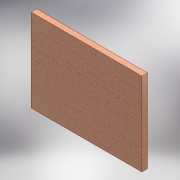
# Autodesk Inventor part: WoodBase
Saved by Autodesk Inventor 2018.2 (Build 222227000, 227)
## iProperties
Created: 2018-03-28
Part Number: WoodBase
Material: Wood (Oak)
Document SubType Name: Modeling
Designer: Muchen He
Density: 0.76 g/cm^3
Appearance: White Oak - Natural Medium Gloss
Author: Muchen He
Autodesk Inventor part; units mm, degrees
ref_plane "YZ Plane" through (0, 0, 0) normal (1, 0, 0) x (0, 1, 0)
ref_plane "XZ Plane" through (0, 0, 0) normal (0, 1, 0) x (-1, 0, 0)
ref_plane "XY Plane" through (0, 0, 0) normal (0, 0, 1) x (1, 0, 0)
sketch "Sketch1" plane through (0, 0, 0) normal (0, 1, 0) x (-1, 0, 0)
  line L0 (0, 0) -> (-400, 0)
  line L1 (-400, 0) -> (-400, -300)
  line L2 (-400, -300) -> (0, -300)
  line L3 (0, -300) -> (0, 0)
  dimension "d0" = 400
  dimension "d1" = 300
  constraints: 8 end point, 2 parallel, 1 horizontal, 1 perpendicular
  measures "d0" distance of L2.end L1.end
  measures "d1" distance of L1.end L0.end
extrude "Extrusion1" add sketch "Sketch1" along normal blind 25.4
chamfer "Chamfer1" distance 5 angle 45 4 edges at (200, 25.4, 0) (400, 25.4, -150) (200, 25.4, -300) (0, 25.4, -150)
body "Solid1"
